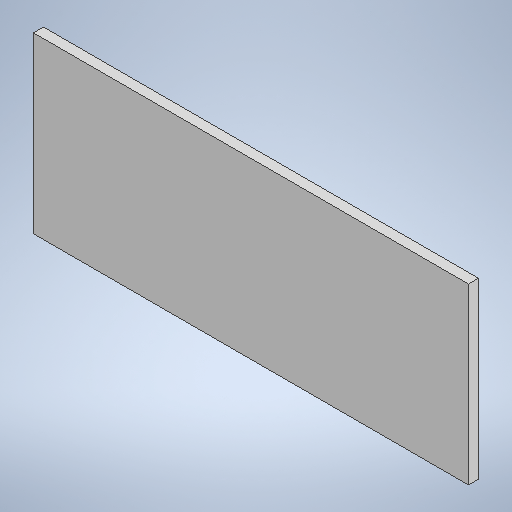
# Autodesk Inventor part: tabla
Saved by Autodesk Inventor 2025.1 (Build 291241000, 241)
## iProperties
Created: 2025-01-11
Part Number: tabla
Material: Generic
Document SubType Name: Modeling
Designer: Hp
Density: 1 g/cm^3
Appearance: Default
Author: Hp
Autodesk Inventor part; units mm, degrees
ref_plane "YZ Plane" through (0, 0, 0) normal (1, 0, 0) x (0, 1, 0)
ref_plane "XZ Plane" through (0, 0, 0) normal (0, 1, 0) x (-1, 0, 0)
ref_plane "XY Plane" through (0, 0, 0) normal (0, 0, 1) x (1, 0, 0)
sketch "Boceto1" plane through (0, 0, 0) normal (0, 0, 1) x (1, 0, 0)
  line L0 (-17.67, 264.8638) -> (16492.33, 264.8638)
  line L1 (16492.33, 264.8638) -> (16492.33, -6339.1362)
  line L2 (16492.33, -6339.1362) -> (-17.67, -6339.1362)
  line L3 (-17.67, -6339.1362) -> (-17.67, 264.8638)
  point P0 (0, 0)
  dimension "d0" = 16510
  dimension "d1" = 6604
  constraints: 8 end point, 2 parallel, 1 horizontal, 1 perpendicular
  measures "d0" distance of L1.end L2.end
  measures "d1" distance of L0.end L1.end
extrude "Extrusión1" add sketch "Boceto1" along normal blind 381
